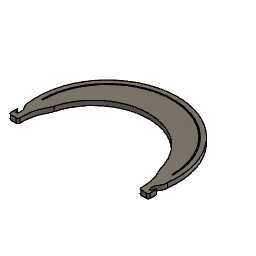
Facemask v3 (Autodesk Fusion 360 design; units mm, degrees)
Autodesk Fusion 360 part; units mm, degrees
sketch "Sketch1" plane through (0, 0, 0) normal (0, 1, 0) x (1, 0, 0)
  arc A0 (90.2509, 0) -> (0, 90.2509) centre (0, 0) ccw
  arc A1 (73.6296, 0) -> (0, 56.5756) centre (0, -19.6244) ccw
  arc A2 (95.4446, -13.0328) -> (0, 96.3326) centre (-0.0015, 0.0007) ccw
  arc A3 (88.9809, 0) -> (0, 88.9809) centre (0, 0) ccw
  line L0 (-90.2509, 0) -> (-88.9809, 0)
  spline S0 degree 5 poles (73.6296, 0) (73.7964, -0.5705) (74.1704, -1.7101) (74.8523, -3.4151) (75.9742, -5.6996) (77.5715, -8.6856) (79.1735, -11.934) (80.6065, -15.5616) (81.7721, -19.6181) (82.6333, -24.103) (83.136, -28.5564) (83.341, -32.2698) (83.3954, -35.0547) (83.3947, -36.7911) (83.3902, -37.4146) knots 0 0 0 0 0 0 0.1 0.2 0.3 0.4 0.5 0.6 0.7 0.8 0.9 0.955263 0.955263 0.955263 0.955263 0.955263 0.955263
  line L1 (72.6061, 3.5011) -> (74.6531, -3.5011)
  line L2 (85.9301, -39.973) -> (93.504, -39.973)
  line L3 (96.044, -37.433) -> (96.044, -28.2682)
  line L4 (95.5671, -28.1465) -> (92.6936, -33.4094)
  line L5 (92.3337, -33.623) -> (90.9425, -33.623)
  spline S1 degree 5 poles (95.4446, -13.0328) (95.4819, -13.3222) (95.539, -13.896) (95.572, -14.7411) (95.51, -15.8369) (95.2545, -17.1547) (94.8261, -18.4229) (94.2408, -19.6479) (93.5335, -20.8429) (92.7609, -22.0288) (91.9906, -23.2304) (91.2921, -24.473) (90.7281, -25.7792) (90.3439, -27.1653) (90.1626, -28.6391) (90.1934, -30.2034) (90.3884, -31.5269) (90.629, -32.5595) (90.831, -33.2655) (90.9425, -33.623) knots 0 0 0 0 0 0 0.066667 0.133333 0.2 0.266667 0.333333 0.4 0.466667 0.533333 0.6 0.666667 0.733333 0.8 0.866667 0.933333 1 1 1 1 1 1
  arc A4 (92.3337, -33.623) -> (92.6936, -33.4094) centre (92.3337, -33.213) ccw
  arc A5 (83.3902, -37.4146) -> (85.9301, -39.973) centre (85.9301, -37.433) ccw
  arc A6 (93.504, -39.973) -> (96.044, -37.433) centre (93.504, -37.433) ccw
  arc A7 (96.044, -28.2682) -> (95.5671, -28.1465) centre (95.79, -28.2682) ccw
  arc A8 (-95.5671, -28.1465) -> (-96.044, -28.2682) centre (-95.79, -28.2682) ccw
  line L6 (-96.044, -37.433) -> (-96.044, -28.2682)
  arc A9 (-85.9301, -39.973) -> (-83.3902, -37.4146) centre (-85.9301, -37.433) ccw
  arc A10 (-96.044, -37.433) -> (-93.504, -39.973) centre (-93.504, -37.433) ccw
  spline S2 degree 5 poles (-95.4446, -13.0328) (-95.4819, -13.3222) (-95.539, -13.896) (-95.572, -14.7411) (-95.51, -15.8369) (-95.2545, -17.1547) (-94.8261, -18.4229) (-94.2408, -19.6479) (-93.5335, -20.8429) (-92.7609, -22.0288) (-91.9906, -23.2304) (-91.2921, -24.473) (-90.7281, -25.7792) (-90.3439, -27.1653) (-90.1626, -28.6391) (-90.1934, -30.2034) (-90.3884, -31.5269) (-90.629, -32.5595) (-90.831, -33.2655) (-90.9425, -33.623) knots 0 0 0 0 0 0 0.066667 0.133333 0.2 0.266667 0.333333 0.4 0.466667 0.533333 0.6 0.666667 0.733333 0.8 0.866667 0.933333 1 1 1 1 1 1
  line L7 (95.1319, -10.6077) -> (95.7573, -15.4579)
  line L8 (90.1321, -31.0241) -> (91.7529, -36.2218)
  line L9 (-95.1319, -10.6077) -> (-95.7573, -15.4579)
  line L10 (-90.1321, -31.0241) -> (-91.7529, -36.2218)
  arc A11 (0, 90.2509) -> (-90.2509, 0) centre (0, 0) ccw
  arc A12 (0, 56.5756) -> (-73.6296, 0) centre (0, -19.6244) ccw
  line L11 (-85.9301, -39.973) -> (-93.504, -39.973)
  spline S3 degree 5 poles (-73.6296, 0) (-73.7964, -0.5705) (-74.1704, -1.7101) (-74.8523, -3.4151) (-75.9742, -5.6996) (-77.5715, -8.6856) (-79.1735, -11.934) (-80.6065, -15.5616) (-81.7721, -19.6181) (-82.6333, -24.103) (-83.136, -28.5564) (-83.341, -32.2698) (-83.3954, -35.0547) (-83.3947, -36.7911) (-83.3902, -37.4146) knots 0 0 0 0 0 0 0.1 0.2 0.3 0.4 0.5 0.6 0.7 0.8 0.9 0.955263 0.955263 0.955263 0.955263 0.955263 0.955263
  line L12 (83.4236, -32.561) -> (83.3568, -42.2681)
  line L13 (-72.6061, 3.5011) -> (-74.6531, -3.5011)
  line L14 (-83.4236, -32.561) -> (-83.3568, -42.2681)
  line L15 (-95.5671, -28.1465) -> (-92.6936, -33.4094)
  arc A13 (0, 88.9809) -> (-88.9809, 0) centre (0, 0) ccw
  arc A14 (0, 96.3326) -> (-95.4446, -13.0328) centre (0.0015, 0.0007) ccw
  line L16 (-92.3337, -33.623) -> (-90.9425, -33.623)
  arc A15 (-92.6936, -33.4094) -> (-92.3337, -33.623) centre (-92.3337, -33.213) ccw
  line L17 (90.2509, 0) -> (88.9809, 0)
  point P0 (79.4459, -12.7634)
  point P1 (83.344, -39.973)
  point P2 (96.044, -39.973)
  point P3 (96.044, -27.273)
  point P4 (90.9399, -25.3534)
  point P5 (94.3711, -19.329)
  point P6 (-83.344, -39.973)
  point P7 (-96.044, -27.273)
  point P8 (-79.4459, -12.7634)
  point P9 (-96.044, -39.973)
  point P10 (-94.3711, -19.329)
  point P11 (-90.9399, -25.3534)
  dimension "d1" = 180.5018
  dimension "d3" = 177.9618
  dimension "d4" = 12.7
  dimension "d5" = 12.7
  dimension "d6" = 0.41
  dimension "d7" = 2.54
  dimension "d8" = 2.54
  dimension "d9" = 0.254
  constraint coincident A0.centre A3.centre
  constraint horizontal L0
  constraint midpoint A1.start L1
  constraint coincident A1 L1.start
  constraint horizontal L2
  constraint perpendicular L2 L3
  constraint perpendicular L3 L5
  constraint tangent L4 A4
  constraint tangent L5 A4
  constraint coincident P1 L2
  constraint tangent S0 A5
  constraint tangent L2 A5
  constraint coincident P2 L2
  constraint coincident P2 L3
  constraint tangent L2 A6
  constraint tangent L3 A6
  constraint coincident P3 L3
  constraint coincident P3 L4
  constraint tangent L3 A7
  constraint tangent L4 A7
  constraint midpoint A2.start L7
  constraint midpoint L5.end L8
  constraint midpoint S0.end L12
  constraint horizontal L17
  measures "d1" diameter of A0
  measures "d3" diameter of A3
  measures "d4" distance of P1 P2
  measures "d5" distance of P2 P3
  measures "d6" radius of A4
  measures "d7" radius of A5
  measures "d8" radius of A6
  measures "d9" radius of A7
extrude "Extrude1" add sketch "Sketch1" along normal blind 6.35 contours A1 A2 S0 L2 L3 L4 L5 S1 A4 A5 A6 A7 A8 L6 A9 A10 S2 A12 L11 S3 L15 A14 L16 A15
equation "d1 = ( ( 22 / 3.14 ) * 1 in ) + 0.1 in"
equation "d3 = ( ( 22 / 3.14 ) * 1 in )"
